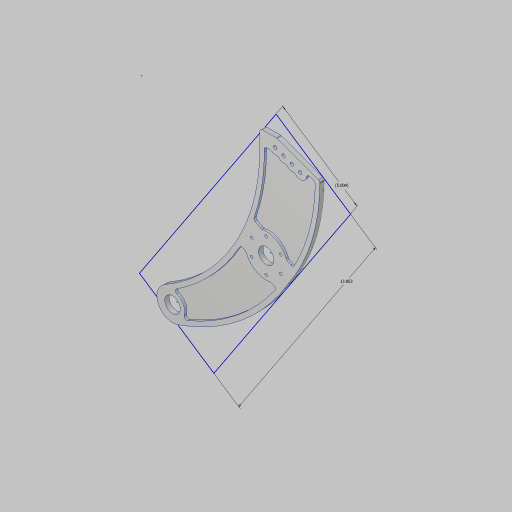
# Autodesk Inventor part: CL7-008
Saved by Autodesk Inventor 2023.5 (Build 275446000, 446)
## iProperties
Created: 2025-03-17
Part Number: CL7-008
Material: Aluminum 6061
Document SubType Name: Modeling
Designer: slick
Density: 2.7 g/cm^3
Appearance: Aluminum - Flat
Mass: 413.954 g
Surface Area: 552.748 cm^2
Volume: 153.316 cm^3
Author: slick
Autodesk Inventor part; units mm, degrees
ref_plane "YZ Plane" through (0, 0, 0) normal (1, 0, 0) x (0, 1, 0)
ref_plane "XZ Plane" through (0, 0, 0) normal (0, 1, 0) x (-1, 0, 0)
ref_plane "XY Plane" through (0, 0, 0) normal (0, 0, 1) x (1, 0, 0)
sketch "Sketch1" plane through (0, 0, 0) normal (0, 0, 1) x (1, 0, 0)
  line L0 (-146.05, 152.4) -> (76.2, 152.4) construction
  line L1 (76.2, 152.4) -> (76.2, 127) construction
  line L2 (76.2, 127) -> (-146.05, 127) construction
  line L3 (-146.05, 127) -> (-146.05, 152.4) construction
  circle A0 centre (-133.35, -127) radius 12.7 construction
  circle A1 centre (0, 0) radius 23.8125 construction
  circle A2 centre (0, 0) radius 11.1125
  circle A3 centre (0, 0) radius 36.5125 construction
  line L4 (76.2, 152.4) -> (76.2, 127)
  line L5 (76.2, 152.4) -> (-9.0845, 152.4)
  line L6 (-9.0845, 152.4) -> (-9.0845, 127)
  circle A4 centre (-133.35, -127) radius 22.225 construction
  arc A5 (-144.4803, -107.7629) -> (-9.0845, 127) centre (-280.3101, 127) ccw
  arc A6 (-126.1231, -148.0172) -> (31.5864, -18.3156) centre (-221.1051, 128.2089) ccw
  arc A7 (-144.4803, -107.7629) -> (-126.1231, -148.0172) centre (-133.35, -127) ccw
  arc A8 (30.0156, -20.79) -> (76.2, 127) centre (-183.3562, 127) ccw
  arc A9 (31.5864, -18.3156) -> (30.9373, -19.3918) centre (0, 0) ccw
  line L7 (-69.85, 152.4) -> (-69.85, 127) construction
  line L8 (12.7, 139.7) -> (75.9941, 116.6628) construction
  line L9 (14.9394, 152.4) -> (76.2, 130.1029)
  point P0 (63.5, 139.7)
  point P1 (76.2, 139.7)
  point P2 (50.8, 139.7)
  point P3 (38.1, 139.7)
  point P4 (25.4, 139.7)
  point P5 (30.0156, -20.79)
  point P6 (-33.2582, 15.0683)
  point P7 (30.851, -19.5766)
  point P8 (-69.85, 139.7)
  point P9 (24.6341, 135.3563)
  point P10 (36.5682, 131.0127)
  point P11 (48.5023, 126.669)
  dimension "d0" = 25.4
  dimension "d1" = 127
  dimension "d2" = 222.25
  dimension "d3" = 146.05
  dimension "d4" = 25.4
  dimension "d5" = 127
  dimension "d7" = 12.7
  dimension "d8" = 47.625
  dimension "d9" = 22.225
  dimension "d12" = 12.7
  dimension "d17" = 12.7
  dimension "d18" = 9.525
  dimension "d19" = 292.1
  dimension "d37" = 146.05
  dimension "d38" = 63.5
  dimension "d39" = 20
  dimension "d42" = 12.7
  dimension "d47" = 12.7
  constraints: 20 end point, 16 point on circle, 10 centre point, 7 tangent, 6 point on line, 5 coincident, 3 parallel, 3 perpendicular, 2 horizontal, 2 midpoint, 1 horizontal alignment, 1 vertical, 8 other
  measures "d0" distance of L2.end L0.start
  measures "d1" distance from line of point (0, 0) L2
  measures "d2" distance of L0.start L0.end
  measures "d3" distance from line of point (0, 0) L3
  measures "d4" diameter of A0
  measures "d5" vertical distance of A0.centre point (0, 0)
  measures "d7" distance from line of L1 point (63.5, 139.7)
  measures "d8" diameter of A1
  measures "d9" diameter of A2
  measures "d12" distance of point (63.5, 139.7) point (50.8, 139.7)
  measures "d17" radial gap between concentric circles of A1 A3
  measures "d18" radial gap between concentric circles of A0 A4
  measures "d19" radius of A6
  measures "d37" distance from line of L0.end L7
  measures "d38" horizontal distance of point (-133.35, -127) point (-69.85, 139.7)
  measures "d39" angle of L2 L8
  measures "d42" distance of L8.start point (24.634, 135.356)
  measures "d47" distance between parallel lines of L8 L9
extrude "Extrusion1" add sketch "Sketch1" along normal blind 6.35 contours L4 A8 A6 A9 A5 L6 L5 L9 | A8 A9 A6 | A6 A7 A5 A9 A8
hole "Hole1" at (36.5682, 131.0127, 0) at (48.5023, 126.669, 0) at (24.6341, 135.3563, 0) at (12.7, 139.7, 0) direction (0, 0, 1) diameter 5.1054 end through all clearance for "Flat Head Machine Screw (82)" size "#10" standard "Ansi Unified Screw Threads"
hole "Hole2" at (-133.35, -127, 0) direction (0, 0, 1) diameter 22.225 end through all
fillet "Fillet1" radius 3.175 3 edges at (76.2, 130.1029, 3.175) (14.9394, 152.4, 3.175) (-9.0845, 152.4, 3.175)
sketch "Sketch3" plane through (0, 0, 6.35) normal (0, 0, 1) x (1, 0, 0)
  arc A0 (-5.9095, 152.4) -> (-9.0845, 149.225) centre (-5.9095, 149.225) ccw construction
  line L0 (-9.0845, 149.225) -> (-9.0845, 127) construction
  arc A1 (-144.4803, -107.7629) -> (-9.0845, 127) centre (-280.3101, 127) ccw construction
  arc A2 (-144.4803, -107.7629) -> (-126.1231, -148.0172) centre (-133.35, -127) ccw construction
  arc A3 (-126.1231, -148.0172) -> (30.851, -19.5766) centre (-221.1051, 128.2089) ccw construction
  arc A4 (30.851, -19.5766) -> (76.2, 127) centre (-183.3562, 127) ccw construction
  line L1 (76.2, 127) -> (76.2, 127.8798) construction
  arc A5 (76.2, 127.8798) -> (74.1109, 130.8633) centre (73.025, 127.8798) ccw construction
  line L2 (74.1109, 130.8633) -> (15.4654, 152.2085) construction
  arc A6 (15.4654, 152.2085) -> (14.3795, 152.4) centre (14.3795, 149.225) ccw construction
  line L3 (14.3795, 152.4) -> (-5.9095, 152.4) construction
  circle A7 centre (-133.35, -127) radius 11.1125 construction
  circle A8 centre (24.6341, 135.3563) radius 2.5527 construction
  circle A9 centre (36.5682, 131.0127) radius 2.5527 construction
  circle A10 centre (48.5023, 126.669) radius 2.5527 construction
  circle A11 centre (12.7, 139.7) radius 2.5527 construction
  circle A12 centre (0, 0) radius 11.1125 construction
  circle A13 centre (0, 0) radius 23.8125 construction
  point P0 (0, 23.8125)
  point P1 (-20.6222, 11.9063)
  point P2 (-20.6222, -11.9062)
  point P3 (0, -23.8125)
  point P4 (20.6222, -11.9063)
  point P5 (20.6222, 11.9062)
  dimension "d49" = 47.625
  dimension "d52" = 360
  constraints: 2 vertical alignment, 1 coincident, 9 other
hole "Hole3" at (0, 23.8125, 6.35) at (-20.6222, 11.9063, 6.35) at (-20.6222, -11.9062, 6.35) at (0, -23.8125, 6.35) at (20.6222, -11.9063, 6.35) at (20.6222, 11.9062, 6.35) direction (0, 0, -1) diameter 3.9624 end through all thread size "10-32 UNF" class "2B" standard "ANSI Unified Screw Threads"
sketch "Sketch4" plane through (0, 0, 6.35) normal (0, 0, 1) x (1, 0, 0)
  circle A0 centre (20.6222, -11.9063) radius 1.9812 construction
  circle A1 centre (-20.6222, -11.9062) radius 1.9812 construction
  circle A2 centre (0, 23.8125) radius 1.9812 construction
  circle A3 centre (-20.6222, 11.9063) radius 1.9812 construction
  circle A4 centre (0, -23.8125) radius 1.9812 construction
  circle A5 centre (20.6222, 11.9062) radius 1.9812 construction
  arc A6 (-5.9095, 152.4) -> (-9.0845, 149.225) centre (-5.9095, 149.225) ccw construction
  line L0 (-9.0845, 149.225) -> (-9.0845, 127) construction
  arc A7 (-144.4803, -107.7629) -> (-9.0845, 127) centre (-280.3101, 127) ccw construction
  arc A8 (-144.4803, -107.7629) -> (-126.1231, -148.0172) centre (-133.35, -127) ccw construction
  arc A9 (-126.1231, -148.0172) -> (30.851, -19.5766) centre (-221.1051, 128.2089) ccw construction
  arc A10 (30.851, -19.5766) -> (76.2, 127) centre (-183.3562, 127) ccw construction
  line L1 (76.2, 127) -> (76.2, 127.8798) construction
  arc A11 (76.2, 127.8798) -> (74.1109, 130.8633) centre (73.025, 127.8798) ccw construction
  line L2 (74.1109, 130.8633) -> (15.4654, 152.2085) construction
  arc A12 (15.4654, 152.2085) -> (14.3795, 152.4) centre (14.3795, 149.225) ccw construction
  line L3 (14.3795, 152.4) -> (-5.9095, 152.4) construction
  circle A13 centre (-133.35, -127) radius 11.1125 construction
  circle A14 centre (24.6341, 135.3563) radius 2.5527 construction
  circle A15 centre (36.5682, 131.0127) radius 2.5527 construction
  circle A16 centre (48.5023, 126.669) radius 2.5527 construction
  circle A17 centre (12.7, 139.7) radius 2.5527 construction
  circle A18 centre (0, 0) radius 11.1125 construction
  circle A19 centre (0, 0) radius 30.1625 construction
  arc A20 (25.4856, -16.173) -> (69.8464, 125.6579) centre (-183.3562, 127) ccw construction
  arc A21 (-128.1879, -142.0123) -> (25.4856, -16.173) centre (-221.1051, 128.2089) ccw construction
  arc A22 (-141.3002, -113.2592) -> (-128.1879, -142.0123) centre (-133.35, -127) ccw construction
  arc A23 (-141.3002, -113.2592) -> (-2.7345, 127) centre (-280.3101, 127) ccw construction
  line L4 (-2.7345, 127) -> (-2.7345, 146.05) construction
  line L5 (-2.7345, 146.05) -> (13.8197, 146.05) construction
  line L6 (69.8464, 125.6579) -> (13.8197, 146.05) construction
  circle A24 centre (12.7, 139.7) radius 8.9027 construction
  circle A25 centre (24.6341, 135.3563) radius 2.5527 construction
  circle A26 centre (24.6341, 135.3563) radius 8.9027 construction
  circle A27 centre (36.5682, 131.0127) radius 8.9027 construction
  circle A28 centre (48.5023, 126.669) radius 8.9027 construction
  circle A29 centre (-133.35, -127) radius 17.4625 construction
  arc A30 (-18.2433, 35.5165) -> (-2.7345, 127) centre (-280.3101, 127) ccw
  arc A31 (38.1257, 4.2843) -> (69.8464, 125.6579) centre (-183.3562, 127) ccw
  arc A32 (-135.2217, -109.6381) -> (-36.2919, -5.3003) centre (-280.3101, 127) ccw
  arc A33 (-121.1415, -139.4856) -> (-135.2217, -109.6381) centre (-133.35, -127) ccw
  line L7 (-18.2433, 35.5165) -> (-7.0656, 29.3233)
  line L8 (38.1257, 4.2843) -> (28.6082, 9.5576)
  line L9 (14.5187, -33.4528) -> (7.0656, -29.3233)
  line L10 (-36.2919, -5.3003) -> (-28.6082, -9.5576)
  arc A34 (-121.1415, -139.4856) -> (14.5187, -33.4528) centre (-221.1051, 128.2089) ccw
  circle A35 centre (0, 0) radius 11.1125 construction
  arc A36 (-28.6082, -9.5576) -> (7.0656, -29.3233) centre (0, 0) ccw
  arc A37 (28.6082, 9.5576) -> (-7.0656, 29.3233) centre (0, 0) ccw
  arc A38 (40.4011, 122.9773) -> (56.5376, 130.5019) centre (48.5023, 126.669) ccw
  arc A39 (28.467, 127.321) -> (40.4011, 122.9773) centre (36.5682, 131.0127) ccw
  arc A40 (16.5329, 131.6646) -> (28.467, 127.321) centre (24.6341, 135.3563) ccw
  arc A41 (6.4602, 133.35) -> (16.5329, 131.6646) centre (12.7, 139.7) ccw
  line L11 (6.4602, 133.35) -> (-2.7345, 133.35)
  line L12 (-2.7345, 133.35) -> (-2.7345, 127)
  line L13 (69.8464, 125.6579) -> (56.5376, 130.5019)
  dimension "d62" = 6.35
  dimension "d63" = 6.35
  dimension "d64" = 6.35
  dimension "d65" = 6.35
  dimension "d66" = 6.35
  dimension "d67" = 6.35
  dimension "d68" = 22.225
  dimension "d69" = 22.225
  dimension "d70" = 12.7
  constraints: 51 point on circle, 21 centre point, 20 end point, 15 coincident, 7 equal radius, 3 parallel, 2 collinear, 2 point on line, 1 line through centre, 1 perpendicular, 1 tangent, 1 vertical, 3 other
  measures "d62" radial gap between concentric circles of A7 A23
  measures "d63" distance between parallel lines of L2 L6
  measures "d64" distance between parallel lines of L3 L5
  measures "d65" radial gap between concentric circles of A10 A20
  measures "d66" radial gap between concentric circles of A17 A24
  measures "d67" radial gap between concentric circles of A13 A29
  measures "d68" distance from line of L10 point (0, 0)
  measures "d69" distance from line of L8 point (0, 0)
  measures "d70" distance between parallel lines of L5 L11
extrude "Extrusion2" cut sketch "Sketch4" against normal blind 3.175
fillet "Fillet2" radius 3.302 17 edges at (-135.2217, -109.6381, 4.7625) (-121.1415, -139.4856, 4.7625) (-36.2919, -5.3003, 4.7625) (-28.6082, -9.5576, 4.7625) (7.0656, -29.3233, 4.7625) (14.5187, -33.4528, 4.7625) (38.1257, 4.2843, 4.7625) (28.6082, 9.5576, 4.7625) (-7.0656, 29.3233, 4.7625) (-18.2433, 35.5165, 4.7625) (-2.7345, 133.35, 4.7625) (6.4602, 133.35, 4.7625) (16.5329, 131.6646, 4.7625) (28.467, 127.321, 4.7625) (40.4011, 122.9773, 4.7625) (56.5376, 130.5019, 4.7625) (69.8464, 125.6579, 4.7625)
sketch "Sketch5" plane through (0, 0, 0) normal (0, 0, -1) x (-1, 0, 0)
  line L0 (-113.4135, 104.9143) -> (81.0094, -188.3634)
  line L1 (81.0094, -188.3634) -> (186.9556, -118.1283)
  line L2 (186.9556, -118.1283) -> (-7.4673, 175.1494)
  line L3 (-7.4673, 175.1494) -> (-113.4135, 104.9143)
  arc A0 (-76.2, 127) -> (-30.851, -19.5766) centre (183.3562, 127) ccw construction
  arc A1 (9.0845, 149.225) -> (5.9095, 152.4) centre (5.9095, 149.225) ccw construction
  arc A2 (126.1231, -148.0172) -> (144.4803, -107.7629) centre (133.35, -127) ccw construction
  arc A3 (-74.1109, 130.8633) -> (-76.2, 127.8798) centre (-73.025, 127.8798) ccw construction
  point P0 (0, 0)
  dimension "d74" = 351.8694
  dimension "d75" = 127.1124
  constraints: 8 end point, 4 tangent, 2 parallel, 1 perpendicular
  measures "d74" distance of L0.start L0.end
  measures "d75" distance of L2.end L0.start
body "Solid1"
